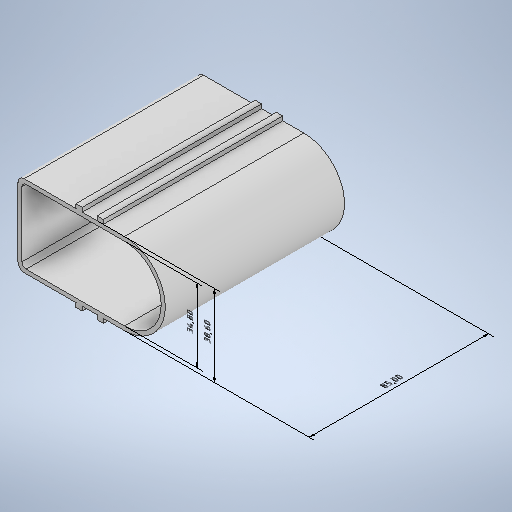
# Autodesk Inventor part: víko
Saved by Autodesk Inventor 2025.3 (Build 293356000, 356)
## iProperties
Created: 2025-06-12
Part Number: víko
Material: Generic
Document SubType Name: Modeling
Designer: Repete
Density: 1 g/cm^3
Appearance: Default
Author: Repete
Autodesk Inventor part; units mm, degrees
ref_plane "YZ Plane" through (0, 0, 0) normal (1, 0, 0) x (0, 1, 0)
ref_plane "XZ Plane" through (0, 0, 0) normal (0, 1, 0) x (-1, 0, 0)
ref_plane "XY Plane" through (0, 0, 0) normal (0, 0, 1) x (1, 0, 0)
sketch "Sketch1" plane through (0, 0, 0) normal (0, 1, 0) x (-1, 0, 0)
  line L0 (35.4, 17.4) -> (35.4, -17.4)
  line L1 (35.4, -17.4) -> (-13.2013, -17.4)
  arc A0 (-13.2013, 17.4) -> (-13.2013, -17.4) centre (-13.2013, 0) ccw
  line L2 (-13.2013, 17.4) -> (35.4, 17.4)
  line L3 (37.3, -19.3) -> (37.3, 19.3)
  line L4 (37.3, 19.3) -> (-13.2013, 19.3)
  arc A1 (-13.2013, 19.3) -> (-13.2013, -19.3) centre (-13.2013, 0) ccw
  line L5 (-13.2013, -19.3) -> (37.3, -19.3)
  point P0 (0, 0)
  point P1 (-13.2013, 0)
  point P2 (0, 0)
  point P3 (-12.8411, -36.7096)
  point P4 (-12.8411, -7.716)
  point P5 (-24.0253, -72.4098)
  constraints: 12 end point, 4 point on circle, 2 centre point, 2 parallel, 2 perpendicular
extrude "Extrusion1" add sketch "Sketch1" along normal blind 83
ref_plane "Work Plane1" through (0, 85, 0) normal (0, 1, 0) x (1, 0, 0)
sketch "Sketch2" plane through (0, 85, 0) normal (0, 1, 0) x (1, 0, 0)
  line L0 (-37.3, 19.3) -> (-37.3, -19.3)
  line L1 (-37.3, -19.3) -> (13.2013, -19.3)
  arc A0 (13.2013, -19.3) -> (13.2013, 19.3) centre (13.2013, 0) ccw
  line L2 (13.2013, 19.3) -> (-37.3, 19.3)
  point P0 (0, 0)
  point P1 (0, 0)
  point P2 (13.2013, 0)
  point P3 (0, 0)
  point P4 (14.0497, 95.3418)
  point P5 (14.0497, 124.3354)
  point P6 (2.8654, 59.6417)
  constraints: 6 end point, 2 point on circle, 1 centre point, 1 parallel, 1 perpendicular
extrude "Extrusion2" add sketch "Sketch2" against normal up to surface (2 mm away)
fillet "Fillet1" radius 3 3 edges at (-37.3, 41.5, -19.3) (-37.3, 84, -19.3) (-37.3, 42.5, 19.3)
fillet "Fillet2" radius 2 2 edges at (-35.4, 41.5, -17.4) (-35.4, 41.5, 17.4)
sketch "Sketch3" plane through (13.2013, 0, -19.3) normal (0, 0, -1) x (-1, 0, 0)
  line L0 (0, 85) -> (47.5013, 85) projected
  line L1 (0, 0) -> (47.5013, 0) projected
  line L2 (10, 85) -> (13, 85)
  line L3 (13, 85) -> (13, 0)
  line L4 (13, 0) -> (10, 0)
  line L5 (10, 0) -> (10, 85)
  line L6 (0, 0) -> (0, 85) projected
  dimension "d28" = 3
  dimension "d29" = 10
  constraints: 8 end point, 2 parallel, 2 point on line, 1 horizontal, 1 perpendicular
  measures "d28" distance between parallel lines of L5 L3
  measures "d29" distance between parallel lines of L6 L5
extrude "Extrusion5" add sketch "Sketch3" along normal blind 2 contours L0 L3 L1 L5
sketch "Sketch8" plane through (-34.3, 0, -19.3) normal (0, 0, -1) x (-1, 0, 0)
  line L0 (0, 85) -> (-47.5013, 85) projected
  line L1 (-34.5013, 0) -> (0, 0) projected
  line L2 (-27.5013, 85) -> (-24.5013, 85)
  line L3 (-24.5013, 85) -> (-24.5013, 0)
  line L4 (-24.5013, 0) -> (-27.5013, 0)
  line L5 (-27.5013, 0) -> (-27.5013, 85)
  line L6 (-34.5013, 0) -> (-34.5013, 85) projected
  point P0 (-34.3, 0)
  dimension "d34" = 7
  dimension "d35" = 3
  constraints: 8 end point, 2 parallel, 2 point on line, 1 horizontal, 1 perpendicular
  measures "d34" distance between parallel lines of L6 L5
  measures "d35" distance between parallel lines of L5 L3
extrude "Extrusion6" add sketch "Sketch8" along normal blind 2 contours L3 L1 L5 L0
sketch "Sketch9" plane through (13.2013, 0, 19.3) normal (0, 0, 1) x (1, 0, 0)
  line L0 (-47.5013, 85) -> (0, 85) projected
  line L1 (-46.6013, 0) -> (0, 0) projected
  line L2 (-13, 85) -> (-10, 85)
  line L3 (-10, 85) -> (-10, 0)
  line L4 (-10, 0) -> (-13, 0)
  line L5 (-13, 0) -> (-13, 85)
  line L6 (0, 0) -> (0, 85) projected
  point P0 (-13.2013, 0)
  dimension "d38" = 10
  dimension "d39" = 3
  constraints: 8 end point, 2 parallel, 2 point on line, 1 horizontal, 1 perpendicular
  measures "d38" distance between parallel lines of L3 L6
  measures "d39" distance between parallel lines of L5 L3
extrude "Extrusion7" add sketch "Sketch9" along normal blind 2 contours L0 L3 L1 L5
sketch "Sketch10" plane through (-34.3, 0, 19.3) normal (0, 0, 1) x (1, 0, 0)
  line L0 (47.5013, 0) -> (0.9, 0) projected
  line L1 (24.5013, 85) -> (0, 85) projected
  line L2 (27.5013, 0) -> (24.5013, 0)
  line L3 (24.5013, 0) -> (24.5013, 85)
  line L4 (24.5013, 85) -> (27.5013, 85)
  line L5 (27.5013, 85) -> (27.5013, 0)
  line L6 (34.5013, 85) -> (34.5013, 0) projected
  point P0 (34.3, 0)
  dimension "d42" = 7
  dimension "d43" = 3
  constraints: 8 end point, 2 parallel, 2 point on line, 1 horizontal, 1 perpendicular
  measures "d42" distance between parallel lines of L6 L5
  measures "d43" distance between parallel lines of L3 L5
extrude "Extrusion8" add sketch "Sketch10" along normal blind 2
body "Solid1"
